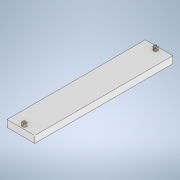
# Autodesk Inventor part: Part6
Saved by Autodesk Inventor 2021 (Build 250183000, 183)
## iProperties
Created: 2021-06-29
Part Number: Part6
Material: LCP Plastic
Document SubType Name: Modeling
Designer: VK
Density: 1.626 g/cm^3
Appearance: Snow
Author: VK
Autodesk Inventor part; units mm, degrees
ref_plane "YZ Plane" through (0, 0, 0) normal (1, 0, 0) x (0, 1, 0)
ref_plane "XZ Plane" through (0, 0, 0) normal (0, 1, 0) x (-1, 0, 0)
ref_plane "XY Plane" through (0, 0, 0) normal (0, 0, 1) x (1, 0, 0)
sketch "Sketch1" plane through (0, 0, 0) normal (0, 1, 0) x (-1, 0, 0)
  line L0 (0, 0) -> (20, 0)
  line L1 (20, 0) -> (20, -100)
  line L2 (20, -100) -> (0, -100)
  line L3 (0, -100) -> (0, 0)
  dimension "d0" = 20
  dimension "d1" = 100
  constraints: 8 end point, 2 parallel, 1 horizontal, 1 perpendicular
  measures "d0" distance of L1.end L2.end
  measures "d1" distance of L0.end L1.end
extrude "Extrusion1" add sketch "Sketch1" along normal blind 5
sketch "Sketch2" plane through (0, 5, 0) normal (0, 1, 0) x (1, 0, 0)
  point P0 (0, 0)
sketch "Sketch3" plane through (0, 5, 0) normal (0, 1, 0) x (1, 0, 0)
  point P0 (0, 0)
sketch "Sketch4" plane through (0, 5, 0) normal (0, 1, 0) x (1, 0, 0)
  point P0 (0, 0)
sketch "Sketch5" plane through (0, 5, 0) normal (0, 1, 0) x (1, 0, 0)
  point P0 (0, 0)
sketch "Sketch6" plane through (0, 5, 0) normal (0, 1, 0) x (1, 0, 0)
  circle A0 centre (-10, 2.5) radius 1.5
  point P0 (0, 0)
  dimension "d4" = 3
  constraints: 1 centre point, 1 coincident
  measures "d4" diameter of A0
extrude "Extrusion2" add sketch "Sketch6" along normal blind 2
sketch "Sketch7" plane through (-10, 7, -2.5) normal (0, 1, 0) x (1, 0, 0)
  line L0 (-0.5, 1.5) -> (0.5, 1.5)
  line L1 (0.5, 1.5) -> (0.5, -1.5)
  line L2 (0.5, -1.5) -> (-0.5, -1.5)
  line L3 (-0.5, -1.5) -> (-0.5, 1.5)
  line L4 (-0.5, 1.5) -> (0.5, -1.5) construction
  line L5 (0.5, 1.5) -> (-0.5, -1.5) construction
  point P0 (10, -2.5)
  point P1 (0, 0)
  dimension "d7" = 1
  dimension "d8" = 3
  constraints: 12 end point, 2 midpoint, 2 parallel, 1 horizontal, 1 perpendicular
  measures "d7" distance of L1.end L2.end
  measures "d8" distance of L0.end L1.end
extrude "Extrusion3" cut sketch "Sketch7" against normal blind 1.5
pattern_linear "Rectangular Pattern1" count 2 spacing 95 along (0, 0, -1) of "Extrusion2", "Extrusion3"
body "Solid1"
